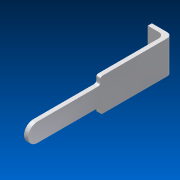
# Autodesk Inventor part: 12mm Incremental Encoder Pin
Saved by Autodesk Inventor 2014 (Build 180170000, 170)
## iProperties
Created: 2011-11-07
Part Number: 12mm Incremental Encoder Pin
Document SubType Name: Modeling
Designer: sdarley
Density: 1 g/cm^3
Material: Generic
Appearance: Polished Brushed
Author: sdarley
Autodesk Inventor part; units mm, degrees
ref_plane "YZ Plane" through (0, 0, 0) normal (1, 0, 0) x (0, 1, 0)
ref_plane "XZ Plane" through (0, 0, 0) normal (0, 1, 0) x (-1, 0, 0)
ref_plane "XY Plane" through (0, 0, 0) normal (0, 0, 1) x (1, 0, 0)
sketch "Sketch1" plane through (0, 0, 0) normal (0, 0, 1) x (1, 0, 0)
  line L0 (0, 0) -> (0.55, 0)
  line L1 (0.8, -0.25) -> (0.8, -6.8)
  line L2 (0.8, -6.8) -> (1, -6.8)
  line L3 (1, -6.8) -> (1, -0.05)
  line L4 (0.75, 0.2) -> (0, 0.2)
  line L5 (0, 0.2) -> (0, 0)
  arc A0 (0.8, -0.25) -> (0.55, 0) centre (0.55, -0.25) ccw
  arc A1 (1, -0.05) -> (0.75, 0.2) centre (0.75, -0.05) ccw
  point P0 (0.8, 0)
  point P1 (1, 0.2)
  dimension "d0" = 0.2
  dimension "d1" = 0.2
  dimension "d2" = 7
  dimension "d3" = 1
  dimension "d6" = 0.25
  constraints: 12 end point, 4 parallel, 4 point on circle, 4 point on line, 4 tangent, 2 centre point, 1 equal radius, 1 horizontal, 1 perpendicular
  measures "d0" distance between parallel lines of L0 L4
  measures "d1" distance between parallel lines of L3 L1
  measures "d2" distance between parallel lines of L2 L4
  measures "d3" distance between parallel lines of L3 L5
  measures "d6" radius of A0
extrude "Extrusion1" add sketch "Sketch1" along normal mid plane 1.6
sketch "Sketch2" plane through (1, -6.8, 0.8) normal (1, 0, 0) x (0, 0, -1)
  line L0 (0, 6.75) -> (0, 0) projected
  line L1 (1.6, 0) -> (0, 0) projected
  line L2 (1.6, 0) -> (1.6, 6.75) projected
  line L3 (0, 3.5) -> (0.35, 3.5)
  line L4 (0.35, 3.5) -> (0.35, 0)
  line L5 (0.35, 0) -> (0, 0)
  line L6 (0, 0) -> (0, 3.5)
  line L7 (1.6, 3.5) -> (1.25, 3.5)
  line L8 (1.25, 3.5) -> (1.25, 0)
  line L9 (1.25, 0) -> (1.6, 0)
  line L10 (1.6, 0) -> (1.6, 3.5)
  point P0 (0.8, 6.8)
  dimension "d8" = 0.9
  dimension "d9" = 3.5
  dimension "d10" = 3.5
  dimension "d11" = 0.35
  constraints: 16 end point, 4 parallel, 4 point on line, 2 horizontal, 2 perpendicular
  measures "d8" distance between parallel lines of L8 L4
  measures "d9" distance between parallel lines of L1 L3
  measures "d10" distance between parallel lines of L1 L7
  measures "d11" distance between parallel lines of L4 L0
extrude "Extrusion2" cut sketch "Sketch2" against normal through all
fillet "Fillet1" radius 0.45 2 edges at (0.9, -6.8, 0.45) (0.9, -6.8, -0.45)
fillet "Fillet2" radius 0.1 4 edges at (0.9, -3.3, 0.8) (0.9, -3.3, 0.45) (0.9, -3.3, -0.45) (0.9, -3.3, -0.8)
equation "\"d1\" = d0"
equation "\"d10\" = d9"
body "Solid1"
